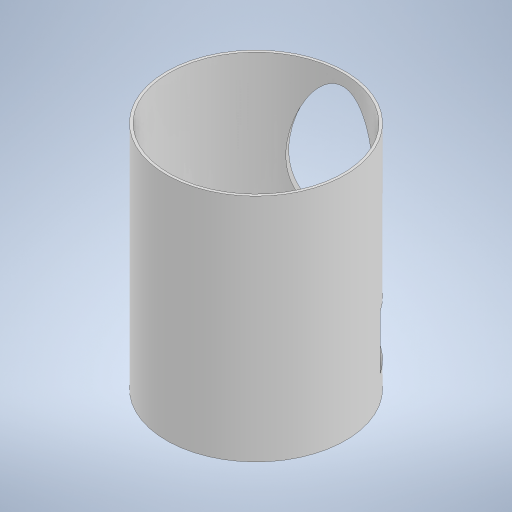
# Autodesk Inventor part: Outer shaft
Saved by Autodesk Inventor 2024.3 (Build 283343000, 343)
## iProperties
Created: 2025-03-01
Part Number: Outer shaft
Material: Generic
Document SubType Name: Modeling
Designer: ajclo
Density: 1 g/cm^3
Appearance: Default
Author: ajclo
Autodesk Inventor part; units mm, degrees
ref_plane "YZ Plane" through (0, 0, 0) normal (1, 0, 0) x (0, 1, 0)
ref_plane "XZ Plane" through (0, 0, 0) normal (0, 1, 0) x (-1, 0, 0)
sketch "Sketch1" plane through (0, 0, 0) normal (0, 1, 0) x (-1, 0, 0)
  circle A0 centre (0, 0) radius 68
  circle A1 centre (0, 0) radius 70
  dimension "d0" = 2
  dimension "d1" = 140
  constraints: 2 centre point, 2 coincident
  measures "d0" radial gap between concentric circles of A1 A0
  measures "d1" diameter of A1
extrude "Extrusion1" add sketch "Sketch1" along normal blind 180
sketch "Sketch2" plane through (0, 0, 0) normal (0, 0, 1) x (1, 0, 0)
  line L0 (-58, 20) -> (58, 20)
  line L1 (58, 20) -> (58, 62)
  line L2 (58, 62) -> (-58, 62)
  line L3 (-58, 62) -> (-58, 20)
  line L4 (70, 0) -> (-70, 0) projected
  point P0 (0, 0)
  point P1 (0, 0)
  dimension "d4" = 42
  dimension "d5" = 116
  dimension "d6" = 20
  dimension "d7" = 58
  constraints: 8 end point, 2 parallel, 1 horizontal, 1 midpoint, 1 perpendicular
  measures "d4" distance of L2.end L0.start
  measures "d5" distance of L1.end L2.end
  measures "d6" distance between parallel lines of L0 L4
  measures "d7" distance from line of L1 point (0, 0)
extrude "Extrusion2" cut sketch "Sketch2" against normal through all
sketch "Sketch3" plane through (0, 0, 0) normal (0, 0, 1) x (1, 0, 0)
  line L0 (32.7477, 110) -> (-36.5, 110)
  line L1 (70, 0) -> (-70, 0) projected
  point P0 (0, 0)
  point P1 (-1.8762, 110)
  dimension "d12" = 110
  constraints: 2 end point, 1 horizontal, 1 midpoint
  measures "d12" distance from line of L1 point (-1.876, 110)
ref_plane "Work Plane1" through (32.7477, 110, 0) normal (0, 0.7071, -0.7071) x (-1, 0, 0)
sketch "Sketch4" plane through (32.7477, 110, 0) normal (0, 0.7071, -0.7071) x (-1, 0, 0)
  circle A0 centre (32.7477, -40) radius 35
  line L0 (0, 0) -> (69.2476, 0) projected
  point P0 (32.7477, -77.7817)
  point P1 (34.6238, 0)
  point P2 (34.6238, 0)
  dimension "d11" = 70
  dimension "d15" = 40
  constraints: 1 centre point, 1 midpoint
  measures "d11" diameter of A0
  measures "d15" vertical distance of A0.centre point (34.624, 0)
extrude "Extrusion3" cut sketch "Sketch4" along normal through all
body "Solid1"
